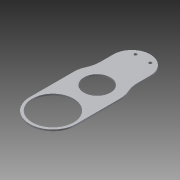
# Autodesk Inventor part: JointC3'cover2_2nd
Saved by Autodesk Inventor 2013 (Build 170138000, 138)
## iProperties
Created: 2013-02-08
Part Number: JointC3'cover2_2nd
Document SubType Name: Modeling
Designer: JohnHenry
Density: 2.71 g/cm^3
Material: アルミニウム 6061
Mass: 3.62463 g
Surface Area: 30.2877 cm^2
Volume: 1.3375 cm^3
Author: JohnHenry
Autodesk Inventor part; units mm, degrees
ref_plane "YZ Plane" through (0, 0, 0) normal (1, 0, 0) x (0, 1, 0)
ref_plane "XZ Plane" through (0, 0, 0) normal (0, 1, 0) x (-1, 0, 0)
ref_plane "XY Plane" through (0, 0, 0) normal (0, 0, 1) x (1, 0, 0)
sketch "スケッチ1" plane through (0, 0, 0) normal (0, 0, 1) x (1, 0, 0)
  circle A0 centre (0, 0) radius 12.5
  circle A1 centre (0, -23.5) radius 15.75
  line L0 (-12.5, 0) -> (-12.5, -13.9181)
  line L1 (12.5, 0) -> (12.5, -13.9181)
  line L2 (0, 0) -> (0, -50.4255)
  point P0 (-15.75, -23.4978)
  point P1 (0.01, 12.5)
  dimension "d0" = 25
  dimension "d1" = 31.5
  dimension "d2" = 23.5
  dimension "d49" = 0
  dimension "d50" = 0
  constraints: 6 end point, 6 point on circle, 2 centre point, 2 tangent, 1 coincident, 1 parallel, 1 vertical
  measures "d0" diameter of A0
  measures "d1" diameter of A1
  measures "d2" distance of A1.centre L2.start
  measures "d49" distance from line of A1.centre L2
  measures "d50" angle of L0 L2
extrude "押し出し2" add sketch "スケッチ1" along normal blind 1
sketch "スケッチ4" plane through (0, 0, 0) normal (0, 0, -1) x (-1, 0, 0)
  arc A0 (12.5, 0) -> (-12.5, 0) centre (0, 0) ccw projected
  point P0 (-5, 7.5)
  point P1 (5, 7.5)
  dimension "d29" = 10
  dimension "d30" = 5
  dimension "d31" = 7.5
  dimension "d32" = 7.5
  measures "d29" distance of point (5, 7.5) point (-5, 7.5)
  measures "d30" horizontal distance of point (5, 7.5) A0.centre
  measures "d31" vertical distance of A0.centre point (5, 7.5)
  measures "d32" vertical distance of A0.centre point (-5, 7.5)
hole "Hole3" at (5, 7.5, 0) at (-5, 7.5, 0) direction (0, 0, 1) diameter 2 depth 8 tip angle 118
sketch "スケッチ5" plane through (0, 0, 0) normal (0, 0, -1) x (-1, 0, 0)
  arc A0 (-12.5, -13.9181) -> (12.5, -13.9181) centre (0, -23.5) ccw projected
  constraints: 1 coincident
hole "Hole4" at (0, -23.5, 0) direction (0, 0, 1) diameter 18 end through all
sketch "スケッチ6" plane through (0, 0, 0) normal (0, 0, -1) x (-1, 0, 0)
  circle A0 centre (0, -23.5) radius 9 projected
  arc A1 (-12.5, -13.9181) -> (12.5, -13.9181) centre (0, -23.5) ccw projected
  line L0 (12.5, 0) -> (12.5, -13.9181) projected
  circle A2 centre (0, -53.5) radius 14
  circle A3 centre (0, -53.5) radius 15.75
  line L1 (-15.75, -23.5) -> (-15.75, -53.5)
  line L2 (15.75, -23.5) -> (15.75, -53.5)
  dimension "d51" = 28
  dimension "d52" = 30
  dimension "d53" = 31.5
  constraints: 4 end point, 4 point on circle, 2 centre point, 2 tangent, 1 coincident, 1 parallel
  measures "d51" diameter of A2
  measures "d52" distance of A2.centre A0.centre
  measures "d53" diameter of A3
extrude "押し出し3" add sketch "スケッチ6" against normal blind 1 contours A1 A3 L1 | A1 A3 | A1 L2 A3 picked at (15.0141, -54.7564)
fillet "フィレット2" radius 20 2 edges at (12.5, -13.9181, 0.5) (-12.5, -13.9181, 0.5)
equation "\"d32\" = d31"
